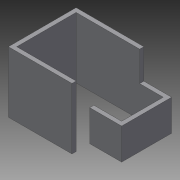
# Autodesk Inventor part: holder
Saved by Autodesk Inventor 2015 (Build 190159000, 159)
## iProperties
Created: 2017-03-02
Part Number: holder
Material: Generic
Document SubType Name: Modeling
Designer: Guy
Density: 1 g/cm^3
Appearance: Default
Author: Guy
Autodesk Inventor part; units mm, degrees
ref_plane "YZ Plane" through (0, 0, 0) normal (1, 0, 0) x (0, 1, 0)
ref_plane "XZ Plane" through (0, 0, 0) normal (0, 1, 0) x (-1, 0, 0)
ref_plane "XY Plane" through (0, 0, 0) normal (0, 0, 1) x (1, 0, 0)
sketch "Sketch4" plane through (0, 0, 0) normal (0, 0, 1) x (1, 0, 0)
  line L0 (0, 0) -> (42.8, 0)
  line L1 (42.8, 0) -> (42.8, 42.8)
  line L2 (42.8, 42.8) -> (0, 42.8)
  line L3 (0, 42.8) -> (0, 0)
  line L4 (-3, 45.8) -> (45.8, 45.8)
  line L5 (45.8, 45.8) -> (45.8, -3)
  line L6 (45.8, -3) -> (-3, -3)
  line L7 (-3, -3) -> (-3, 45.8)
  dimension "d26" = 42.8
  dimension "d27" = 42.8
  dimension "d28" = 3
  constraints: 16 end point, 4 parallel, 2 perpendicular, 1 horizontal, 3 other
  measures "d26" distance of L2.end L1.end
  measures "d27" distance of L0.end L1.end
  measures "d28" distance between parallel lines of L2 L4
extrude "Extrusion6" add sketch "Sketch4" along normal blind 44
sketch "Sketch5" plane through (45.8, -3, 0) normal (1, 0, 0) x (0, 0, -1)
  line L0 (-44, 45.8) -> (0, 45.8)
  line L1 (0, 45.8) -> (0, 0)
  line L2 (0, 0) -> (-44, 0)
  line L3 (-44, 0) -> (-44, 45.8)
  point P0 (0, 3)
  constraints: 8 end point, 2 parallel, 1 coincident, 1 horizontal, 1 perpendicular
extrude "Extrusion7" cut sketch "Sketch5" against normal blind 3
sketch "Sketch6" plane through (45.8, 42.8, 0) normal (1, 0, 0) x (0, 0, -1)
  line L0 (-44, 0) -> (0, 0) projected
  line L1 (0, 3) -> (-22.5, 3)
  line L2 (-22.5, 3) -> (-22.5, 0)
  line L3 (-22.5, 0) -> (0, 0)
  line L4 (0, 0) -> (0, 3)
  point P0 (0, -42.8)
  dimension "d33" = 22.5
  constraints: 8 end point, 2 parallel, 1 horizontal, 1 perpendicular, 1 point on line
  measures "d33" distance between parallel lines of L2 L4
extrude "Extrusion8" add sketch "Sketch6" along normal blind 17
sketch "Sketch7" plane through (62.8, 42.8, 0) normal (1, 0, 0) x (0, 0, -1)
  line L0 (-22.5, 3) -> (0, 3)
  line L1 (0, 3) -> (0, -33)
  line L2 (0, -33) -> (-22.5, -33)
  line L3 (-22.5, -33) -> (-22.5, 3)
  point P0 (0, -42.8)
  dimension "d37" = 36
  constraints: 8 end point, 2 coincident, 2 parallel, 1 horizontal, 1 perpendicular
  measures "d37" distance between parallel lines of L2 L0
extrude "Extrusion9" add sketch "Sketch7" along normal blind 3
sketch "Sketch8" plane through (62.8, 42.8, 0) normal (-1, 0, 0) x (0, 0, 1)
  line L0 (22.5, 0) -> (0, 0) projected
  line L1 (0, 0) -> (0, -33) projected
  line L2 (0, -33) -> (22.5, -33) projected
  line L3 (22.5, -33) -> (22.5, 0) projected
  line L4 (0, -33) -> (22.5, -33)
  line L5 (22.5, -33) -> (22.5, -30)
  line L6 (22.5, -30) -> (0, -30)
  line L7 (0, -30) -> (0, -33)
  point P0 (0, -42.8)
  dimension "d40" = 3
  constraints: 8 end point, 2 parallel, 1 horizontal, 1 perpendicular, 1 point on line
  measures "d40" distance between parallel lines of L2 L6
extrude "Extrusion10" add sketch "Sketch8" along normal blind 20 contours L3 L2 L1 L6
body "Solid3"
